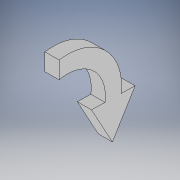
# Autodesk Inventor part: Arrow
Saved by Autodesk Inventor 2018 (Build 220112000, 112)
## iProperties
Created: 2019-01-08
Part Number: Arrow
Material: Generic
Document SubType Name: Modeling
Designer: Gabriel
Density: 1 g/cm^3
Appearance: Default
Author: Gabriel
Autodesk Inventor part; units mm, degrees
ref_plane "YZ Plane" through (0, 0, 0) normal (1, 0, 0) x (0, 1, 0)
ref_plane "XZ Plane" through (0, 0, 0) normal (0, 1, 0) x (-1, 0, 0)
ref_plane "XY Plane" through (0, 0, 0) normal (0, 0, 1) x (1, 0, 0)
sketch "Sketch1" plane through (0, 0, 0) normal (1, 0, 0) x (0, 1, 0)
  line L0 (-25.3272, 15.7999) -> (43.5881, 53.4579)
  line L1 (43.5881, 53.4579) -> (41.7432, -25.0535)
  line L2 (41.7432, -25.0535) -> (-25.3272, 15.7999)
  arc A0 (42.3319, 0) -> (150.3078, 111.7735) centre (53.869, 96.8953) ccw
  arc A1 (43.0157, 29.0986) -> (119.4561, 111.7735) centre (52.6501, 96.8661) ccw
  line L3 (119.4561, 111.7735) -> (150.3078, 111.7735)
  point P0 (0, 0)
  point P1 (20.0014, 14.7347)
  constraints: 8 end point, 4 point on circle, 2 centre point, 2 point on line, 1 horizontal, 7 other
extrude "Extrusion1" add sketch "Sketch1" along normal blind 25.4
body "Solid1"
